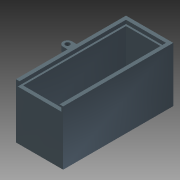
# Autodesk Inventor part: Lead Box
Saved by Autodesk Inventor 2015 (Build 190159000, 159)
## iProperties
Created: 2015-03-10
Part Number: Lead Box
Material: Lead
Document SubType Name: Modeling
Designer: pltwe4
Density: 11.34 g/cm^3
Appearance: Lead
Author: pltwe4
Autodesk Inventor part; units mm, degrees
ref_plane "YZ Plane" through (0, 0, 0) normal (1, 0, 0) x (0, 1, 0)
ref_plane "XZ Plane" through (0, 0, 0) normal (0, 1, 0) x (-1, 0, 0)
ref_plane "XY Plane" through (0, 0, 0) normal (0, 0, 1) x (1, 0, 0)
sketch "Sketch1" plane through (0, 0, 0) normal (0, 0, 1) x (1, 0, 0)
  circle A0 centre (0, 0) radius 14.925 construction
  line L0 (-5.7359, -22.925) -> (4.2584, -22.925) construction
  line L1 (0, -14.925) -> (3.9694, -14.925) construction
  line L2 (-17.5, 17.075) -> (17.5, 17.075)
  line L3 (17.5, 17.075) -> (17.5, -22.925)
  line L4 (17.5, -22.925) -> (-17.5, -22.925)
  line L5 (-17.5, -22.925) -> (-17.5, 17.075)
  line L6 (0, 31.425) -> (0, -35.6875) projected
  line L7 (20.675, 21.8375) -> (20.675, -26.1)
  line L8 (20.675, -26.1) -> (-20.675, -26.1)
  line L9 (-20.675, -26.1) -> (-20.675, 21.8375)
  line L10 (-17.5, 17.075) -> (-19.0875, 17.075)
  line L11 (-19.0875, 17.075) -> (-19.0875, 20.25)
  line L12 (17.5, 17.075) -> (19.0875, 17.075)
  line L13 (19.0875, 17.075) -> (19.0875, 20.25)
  line L14 (17.5, 20.25) -> (17.5, 21.8375)
  line L15 (-17.5, 20.25) -> (-17.5, 21.8375)
  line L16 (-19.0875, 20.25) -> (-17.5, 20.25)
  line L17 (-17.5, 21.8375) -> (-20.675, 21.8375)
  line L18 (19.0875, 20.25) -> (17.5, 20.25)
  line L19 (17.5, 21.8375) -> (20.675, 21.8375)
  line L20 (-17.5, 21.8375) -> (17.5, 21.8375)
  dimension "d0" = 29.85
  dimension "d1" = 8
  dimension "d2" = 40
  dimension "d3" = 35
  dimension "d5" = 3.175
  dimension "d6" = 3.175
  dimension "d7" = 3.175
  dimension "d10" = 3.175
  dimension "d11" = 1.5875
  dimension "d12" = 1.5875
  constraints: 40 end point, 10 horizontal, 3 parallel, 2 collinear, 1 coincident, 1 perpendicular, 1 point on line, 1 vertical alignment, 7 other
  measures "d1" distance between parallel lines of L0 L1
  measures "d2" distance between parallel lines of L4 L2
  measures "d3" distance between parallel lines of L5 L3
  measures "d5" distance between parallel lines of L9 L5
  measures "d6" distance between parallel lines of L8 L4
  measures "d7" distance between parallel lines of L7 L3
  measures "d10" distance between parallel lines of L10 L16
  measures "d11" distance between parallel lines of L9 L11
  measures "d12" distance between parallel lines of L17 L16
extrude "Extrusion1" add sketch "Sketch1" against normal blind 90 contours L5 L4 L6 L8 L9 L17 L15 L16 L11 L10 | L12 L13 L18 L14 L19 L7 L8 L6 L4 L3
extrude "Extrusion2" add sketch "Sketch1" along normal blind 3.175 contours L2 L6 L4 L5 | L5 L4 L6 L8 L9 L17 L15 L16 L11 L10 | L2 L3 L4 L6 | L12 L13 L18 L14 L19 L7 L8 L6 L4 L3
sketch "Sketch2" plane through (0, 0, -90) normal (0, 0, -1) x (-1, 0, 0)
  line L0 (19.0875, 17.075) -> (17.5, 17.075) projected
  line L1 (17.5, 17.075) -> (17.5, -22.925) projected
  line L2 (17.5, -22.925) -> (-17.5, -22.925) projected
  line L3 (-17.5, -22.925) -> (-17.5, 17.075) projected
  line L4 (-17.5, 17.075) -> (-19.0875, 17.075) projected
  line L5 (-19.0875, 17.075) -> (-19.0875, 20.25) projected
  line L6 (-19.0875, 20.25) -> (-17.5, 20.25) projected
  line L7 (-17.5, 20.25) -> (-17.5, 21.8375) projected
  line L8 (-17.5, 21.8375) -> (-20.675, 21.8375) projected
  line L9 (-20.675, 21.8375) -> (-20.675, -26.1) projected
  line L10 (-20.675, -26.1) -> (20.675, -26.1) projected
  line L11 (20.675, -26.1) -> (20.675, 21.8375) projected
  line L12 (20.675, 21.8375) -> (17.5, 21.8375) projected
  line L13 (17.5, 21.8375) -> (17.5, 20.25) projected
  line L14 (17.5, 20.25) -> (19.0875, 20.25) projected
  line L15 (19.0875, 20.25) -> (19.0875, 17.075) projected
  line L16 (-17.5, 21.8375) -> (17.5, 21.8375)
  line L17 (-17.5, 20.25) -> (17.5, 20.25)
  line L18 (-17.5, 17.075) -> (17.5, 17.075)
  point P0 (0, 0)
  constraints: 6 end point, 3 horizontal
extrude "Extrusion3" add sketch "Sketch2" along normal blind 3.175
extrude "Extrusion4" cut sketch "Sketch2" along normal blind 1.5875 contours L0 L18 L4 L5 L6 L17 L14 L15
sketch "Sketch3" plane through (-17.5, -22.925, 0) normal (0, 1, 0) x (1, 0, 0)
  line L0 (-3.175, 93.175) -> (-3.175, -3.175) projected
  line L1 (38.175, 93.175) -> (-3.175, 93.175) projected
  line L2 (38.175, 93.175) -> (38.175, -3.175) projected
  line L3 (-3.175, -3.175) -> (38.175, -3.175) projected
  line L4 (-3.175, 93.175) -> (-3.175, -3.175) construction
  line L5 (-3.175, 45) -> (38.175, 45) construction
  line L6 (38.175, 93.175) -> (38.175, -3.175) construction
  line L7 (-3.175, -3.175) -> (38.175, -3.175) construction
  line L8 (17.5, -3.175) -> (17.5, 93.175) construction
  line L9 (38.175, 93.175) -> (-3.175, 93.175) construction
  circle A0 centre (17.5, 46.03) radius 9.75
  circle A1 centre (17.5, 46.03) radius 12.75 construction
  line L10 (17.5, 58.78) -> (17.5, 55.78) construction
  line L11 (17.5, 57.28) -> (18.611, 57.28) construction
  point P0 (17.5, 0)
  dimension "d22" = 19.5
  dimension "d23" = 25.5
  dimension "d21" = 1.03
  constraints: 8 end point, 5 midpoint, 3 point on line, 2 coincident, 2 vertical alignment, 1 horizontal, 4 other
  measures "d21" distance from line of point (17.5, 46.03) L5
extrude "Extrusion5" cut sketch "Sketch3" against normal up to next contours A0
hole "Hole1" at (0, -22.925, -57.28) direction (0, -1, 0) diameter 2 depth 8 tip angle 118
ref_plane "Work Plane1" through (0, -22.925, 3.175) normal (1, 0, 0) x (0, 0, -1)
ref_plane "Work Plane2" through (-20.675, -22.925, -45) normal (0, 0, -1) x (1, 0, 0)
pattern_circular "Circular Pattern1" count 8 over 360 about axis through (0, -26.1, -46.03) along (0, 1, 0) of "Hole1"
sketch "Sketch4" plane through (-17.5, 21.8375, -90) normal (0, 1, 0) x (1, 0, 0)
  circle A0 centre (25.455, -36.015) radius 1 projected
  circle A1 centre (28.75, -43.97) radius 1 projected
  circle A2 centre (25.455, -51.925) radius 1 projected
  circle A3 centre (17.5, -55.22) radius 1 projected
  circle A4 centre (9.545, -51.925) radius 1 projected
  circle A5 centre (6.25, -43.97) radius 1 projected
  circle A6 centre (9.545, -36.015) radius 1 projected
  circle A7 centre (17.5, -32.72) radius 1 projected
  circle A8 centre (17.5, -43.97) radius 9.75 projected
  line L0 (35, -90) -> (0, -90) projected
  line L1 (35, -90) -> (35, 0) projected
  line L2 (0, 0) -> (35, 0) projected
  line L3 (0, -90) -> (0, 0) projected
  line L4 (0, 0) -> (0, -93.175) projected
  line L5 (0, 0) -> (35, 0) projected
  line L6 (35, 0) -> (35, -93.175) projected
  line L7 (38.175, -93.175) -> (35, -93.175) projected
  line L8 (38.175, 3.175) -> (38.175, -93.175) projected
  line L9 (-3.175, 3.175) -> (38.175, 3.175) projected
  line L10 (-3.175, 3.175) -> (-3.175, -93.175) projected
  line L11 (0, -93.175) -> (-3.175, -93.175) projected
  circle A9 centre (-7.175, -43.97) radius 2
  line L12 (17.5, -43.97) -> (-7.175, -43.97) construction
  arc A10 (-7.175, -39.97) -> (-7.175, -47.97) centre (-7.175, -43.97) ccw
  line L13 (-7.175, -47.97) -> (-3.175, -47.97)
  line L14 (-7.175, -39.97) -> (-3.175, -39.97)
  line L15 (-3.175, 3.175) -> (-3.175, -93.175) projected
  point P0 (17.5, -90)
  dimension "d38" = 4
  dimension "d39" = 4
  dimension "d40" = 2
  constraints: 6 end point, 2 centre point, 2 point on circle, 2 point on line, 2 tangent, 1 coincident, 1 horizontal, 1 parallel, 1 perpendicular
  measures "d38" diameter of A9
  measures "d39" distance from line of L10 L12.end
  measures "d40" radial gap between concentric circles of A9 A10
extrude "Extrusion6" add sketch "Sketch4" against normal blind 5 contours L13 A10 L14 L10
equation "\"d5\" = d4"
equation "\"d6\" = d4"
equation "\"d7\" = d4"
equation "\"d12\" = d11"
equation "\"d4\" = 3.175"
body "Solid1"
